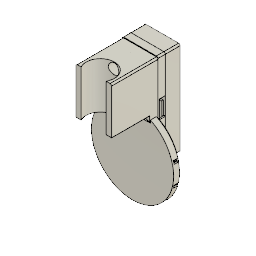
Wall Case v1 (Autodesk Fusion 360 design; units mm, degrees)
Autodesk Fusion 360 part; units mm, degrees
note: some values were not read from the file. Chosen so that the rebuilt part matches the saved one: which face or edge a step refers to. Set by a fixed rule: which sketch regions a step uses.
sketch "Bottom" plane through (0, 0, 0) normal (0, 0, 1) x (1, 0, 0) in component "Coil Case"
  arc A0 (33.9349, 0) -> (34.9349, 1) centre (33.9349, 1) ccw
  arc A1 (34.9349, 23) -> (33.9349, 24) centre (33.9349, 23) ccw
  line L0 (3.9349, 24) -> (3.9349, 0)
  circle A2 centre (30.9349, 12) radius 3.5
  circle A3 centre (30.9349, 12) radius 2.5
  line L1 (0, 0) -> (33.9349, 0)
  line L2 (34.9349, 1) -> (34.9349, 23)
  line L3 (33.9349, 24) -> (0, 24)
  line L4 (30.9349, 12) -> (34.9349, 12) construction
  line L5 (0, 0) -> (0, 24) construction
  circle A4 centre (-23.5651, 12) radius 26.5
  line L6 (0, 12) -> (-23.5651, 12) construction
  circle A5 centre (-23.5651, 12) radius 25.5
  circle A6 centre (-23.5651, 12) radius 2.5
  line L7 (-23.5651, 12) -> (-23.5651, -14.5) construction
  line L8 (-17.5651, -13.8118) -> (-17.5651, -12.7841)
  line L9 (-15.5651, -13.2636) -> (-15.5651, -12.2126)
  line L10 (-29.5651, -13.8118) -> (-29.5651, -12.7841)
  line L11 (-31.5651, -13.2636) -> (-31.5651, -12.2126)
  dimension "d2" = 7
  dimension "d4" = 33.9349
  dimension "d6" = 5
  dimension "d8" = 4
  dimension "d9" = 22
  dimension "d10" = 1
  dimension "d11" = 1
  dimension "d21" = 12
  dimension "d22" = 33.9349
  dimension "d23" = 3.9349
  dimension "d27" = 53
  dimension "d28" = 23.5651
  dimension "d29" = 51
  dimension "d30" = 5
  dimension "d37" = 2
  dimension "d38" = 6
  dimension "d24" = 0
  dimension "d25" = 0
  dimension "d26" = 0
  dimension "d35" = 0
  measures "d2" diameter of A2
  measures "d4" distance of A1.end L3.end
  measures "d6" diameter of A3
  measures "d8" distance of A2.centre L4.end
  measures "d9" distance of A0.end A1.start
  measures "d10" radius of A0
  measures "d11" radius of A1
  measures "d21" distance of A2.centre L1
  measures "d22" distance of A0.start L1.start
  measures "d23" distance of L0 L5
  measures "d27" diameter of A4
  measures "d28" distance of L6.start A4.centre
  measures "d29" diameter of A5
  measures "d30" diameter of A6
  measures "d37" distance of L8 L9
  measures "d38" distance of L7 L8
extrude "Extrude1" add sketch "Bottom" along normal blind 5.5 contours A0 A1 L0 L1 L2 L3 | L0 L1 L3 A4 | A2 makes body 1 in component "Coil Case"
extrude "Extrude2" add sketch "Bottom" along normal blind 25.5 from surface at 5.5 contours A0 A1 L0 L1 L2 L3 bodies 1 in component "Coil Case"
sketch "Side" plane through (34.9349, 0, 0) normal (1, 0, 0) x (0, 1, 0) in component "Coil Case"
  line L0 (1, 0) -> (23, 0)
  line L1 (23, 0) -> (23, 31)
  line L2 (23, 31) -> (1, 31)
  line L3 (1, 31) -> (1, 0)
  line L4 (12, 0) -> (12, 17) construction
  line L5 (12, 17) -> (12, 26.5) construction
  circle A0 centre (12, 26.5) radius 9.5
  dimension "d17" = 17
  dimension "d18" = 9.5
  measures "d17" distance of L4.start L4.end
  measures "d18" distance of L4.end L5.end
extrude "Extrude3" cut sketch "Side" against normal blind 31 contours L2 A0 | L2 A0 bodies 1 in component "Coil Case"
extrude "Extrude4" add sketch "Bottom" along normal blind 1 contours A4 A5 L9 L11 | A4 A5 L8 L9 | A4 A5 L10 L11 | A4 A5 L8 L10 | A5 bodies 1 in component "Coil Case"
extrude "Extrude5" add sketch "Bottom" along normal blind 2 contours A4 A5 L9 L11 | A4 A5 L8 L9 | A4 A5 L10 L11 | A4 A5 L8 L10 bodies 1 in component "Coil Case"
extrude "Extrude6" cut sketch "Bottom" against normal up to surface (1 mm away) from surface at 2 contours A4 A5 L8 L9 | A4 A5 L10 L11 bodies 1 in component "Coil Case"
sketch "Bottom (2)" plane through (0, 0, 0) normal (0, 1, 0) x (-1, 0, 0) in component "Coil Top"
  circle A0 centre (0, 0) radius 26.575
  circle A1 centre (0, 0) radius 27.575
  line L0 (6, -25.8888) -> (6, -26.9143)
  line L1 (8, -26.389) -> (8, -25.3423)
  line L2 (0, 0) -> (0, -27.575) construction
  line L3 (-6, -25.8888) -> (-6, -26.9143)
  line L4 (-8, -26.389) -> (-8, -25.3423)
  line L5 (0, 0) -> (0, 27.575) construction
  line L6 (0, 0) -> (-27.575, 0) construction
  line L7 (-23, 0) -> (-23, 12)
  line L8 (-23, 12) -> (-24.827, 12)
  line L9 (-23, 0) -> (-23, -12)
  line L10 (-23, -12) -> (-24.827, -12)
  dimension "d17_1" = 53.15
  dimension "d18_1" = 55.15
  dimension "d29_1" = 6
  dimension "d30_1" = 2
  dimension "d1" = 0
  dimension "d3" = 0
  dimension "d5" = 0
  dimension "d7" = 0
  dimension "d47" = 12
  dimension "d48" = 12
  measures "d17_1" diameter of A0
  measures "d18_1" diameter of A1
  measures "d29_1" distance of L0 L2
  measures "d30_1" distance of L0 L1
  measures "d47" distance of L7.start L7.end
  measures "d48" distance of L7.start L9.end
extrude "Extrude4'" add sketch "Bottom (2)" along normal blind 1 separate body contours A0 L7 L8 L9 L10 | A0 A1 L4 L10 | A0 A1 L3 L4 | A0 A1 L0 L3 | A0 A1 L0 L1 | A0 A1 L1 L8 picked at (9.9525, 1.3107) makes body 2 in component "Coil Top"
extrude "Extrude5'" add sketch "Bottom (2)" along normal blind 4 contours A0 A1 L4 L10 | A0 A1 L0 L3 | A0 A1 L1 L8 bodies 2 in component "Coil Top"
sketch "Bottom (3)" plane through (0, 0, 0) normal (0, 1, 0) x (-1, 0, 0) in component "PCB Top"
  arc A0 (-1, -24) -> (0, -23) centre (-1, -23) ccw
  line L0 (0, -23) -> (0, -1)
  arc A1 (0, -1) -> (-1, 0) centre (-1, -1) ccw
  line L1 (-63, -23) -> (-63, -1)
  line L2 (0, -1) -> (0, -23)
  arc A2 (-1, -24) -> (0, -23) centre (-1, -23) ccw
  arc A3 (-63, -23) -> (-62, -24) centre (-62, -23) ccw
  arc A4 (-62, 0) -> (-63, -1) centre (-62, -1) ccw
  arc A5 (0, -1) -> (-1, 0) centre (-1, -1) ccw
  circle A6 centre (-59, -12) radius 2.35
  circle A7 centre (-59, -12) radius 1.75
  circle A8 centre (-4, -12) radius 2.35
  circle A9 centre (-4, -12) radius 1.75
  line L3 (-1, -24) -> (-62, -24)
  line L4 (-9.2, -22.7) -> (-9.2, -18.7)
  line L5 (-9.2, -18.7) -> (-11.8, -18.7)
  line L6 (-11.8, -18.7) -> (-11.8, -22.7)
  line L7 (-11.8, -22.7) -> (-25.7, -22.7)
  line L8 (-25.7, -22.7) -> (-25.7, -22.5907)
  line L9 (-25.7, -22.5907) -> (-25.7, -18.7)
  line L10 (-25.7, -18.7) -> (-28.3, -18.7)
  line L11 (-28.3, -18.7) -> (-28.3, -22.7)
  line L12 (-28.3, -22.7) -> (-54.7, -22.7)
  line L13 (-54.7, -22.7) -> (-54.7, -3)
  arc A10 (-54, -2.3) -> (-54.7, -3) centre (-54, -3) ccw
  line L14 (-54, -2.3) -> (-37.3, -2.3)
  line L15 (-37.3, -4.8) -> (-37.3, -2.3)
  line L16 (-24.7, -4.8) -> (-37.3, -4.8)
  line L17 (-24.7, -2.3) -> (-24.7, -4.8)
  line L18 (-24.7, -2.3) -> (-9, -2.3)
  arc A11 (-8.3, -3) -> (-9, -2.3) centre (-9, -3) ccw
  line L19 (-8.3, -3) -> (-8.3, -22.7)
  line L20 (-8.3, -22.7) -> (-9.2, -22.7)
  line L21 (-4, -12) -> (0, -12) construction
  line L22 (-4, -12) -> (-4, 0) construction
  line L23 (-59, -12) -> (-59, 0) construction
  line L24 (-59, -12) -> (-63, -12) construction
  line L25 (-1, 0) -> (-62, 0)
  line L26 (0, 0) -> (-1, 0) construction
  line L27 (0, 0) -> (0, -1) construction
  dimension "d55_1" = 1
  dimension "d61" = 4.7
  dimension "d62" = 3.5
  dimension "d64" = 4.7
  dimension "d65" = 3.5
  dimension "d80" = 12
  dimension "d81" = 4
  dimension "d82" = 61
  dimension "d84" = 22
  dimension "d85" = 12
  dimension "d86" = 4
  dimension "d87" = 61
  dimension "d88" = 1
  dimension "d89" = 2.3
  dimension "d90" = 2.5
  dimension "d91" = 12.6
  dimension "d92" = 2.5
  dimension "d93" = 16.7
  dimension "d94" = 19.7
  dimension "d95" = 0.9
  dimension "d96" = 2.6
  dimension "d97" = 4
  dimension "d98" = 4
  dimension "d99" = 13.9
  dimension "d100" = 3.8907
  dimension "d101" = 2.6
  dimension "d102" = 4
  dimension "d103" = 26.4
  dimension "d104" = 19.7
  dimension "d105" = 0.7
  dimension "d106" = 8.3
  measures "d55_1" radius of A2
  measures "d61" diameter of A6
  measures "d62" diameter of A7
  measures "d64" diameter of A8
  measures "d65" diameter of A9
  measures "d80" distance of A8.centre L22.end
  measures "d81" distance of A8.centre L21.end
  measures "d82" distance of A3.end A0.start
  measures "d84" distance of L1.start L1.end
  measures "d85" distance of A6.centre L23.end
  measures "d86" distance of A6.centre L24.end
  measures "d87" distance of A4.start A1.end
  measures "d88" distance of A1.end L26.start
  measures "d89" distance of L18 L25
  measures "d90" distance of L16.start L17.start
  measures "d91" distance of L15.start L16.start
  measures "d92" distance of L14.end L15.start
  measures "d93" distance of A10.start L14.end
  measures "d94" distance of A11.start L19.end
  measures "d95" distance of L4.start L19.end
  measures "d96" distance of L4.end L5.end
  measures "d97" distance of L4.start L4.end
  measures "d98" distance of L5.end L6.end
  measures "d99" distance of L6.end L7.end
  measures "d100" distance of L8.end L9.end
  measures "d101" distance of L9.end L10.end
  measures "d102" distance of L10.end L11.end
  measures "d103" distance of L11.end L12.end
  measures "d104" distance of L12.end L13.end
  measures "d105" radius of A10
  measures "d106" distance of L2 L19
extrude "Extrude15" add sketch "Bottom (3)" along normal blind 10 separate body contours A0 L0 A1 L1 L2 A2 A3 A4 A5 L3 L25 | A6 | A8 | L4 L5 L6 L7 L8 L9 L10 L11 L12 L13 A10 L14 L15 L16 L17 L18 A11 L19 L20 makes body 3 in component "PCB Top"
extrude "Extrude16" add sketch "Bottom (3)" along normal blind 1 from surface at 10 contours L4 L5 L6 L7 L8 L9 L10 L11 L12 L13 A10 L14 L15 L16 L17 L18 A11 L19 L20 bodies 3 in component "PCB Top"
extrude "Extrude17" add sketch "Bottom (3)" along normal blind 2.5 from surface at 10 contours A6 | A8 bodies 3 in component "PCB Top"
sketch "Bottom (4)" plane through (0, 0, 0) normal (0, 1, 0) x (1, 0, 0) in component "PCB Bottom"
  line L0 (63, 1) -> (63, 23)
  arc A0 (63, 23) -> (62, 24) centre (62, 23) ccw
  arc A1 (62, 0) -> (63, 1) centre (62, 1) ccw
  line L1 (1, 0) -> (62, 0)
  line L2 (8, 23) -> (55, 23)
  circle A2 centre (59, 12) radius 2.5
  line L3 (62, 24) -> (1, 24)
  line L4 (0, 23) -> (0, 1)
  arc A3 (1, 24) -> (0, 23) centre (1, 23) ccw
  arc A4 (0, 1) -> (1, 0) centre (1, 1) ccw
  circle A5 centre (4, 12) radius 2.5
  line L5 (8, 23) -> (8, 3)
  line L6 (55, 23) -> (55, 3)
  line L7 (9, 2) -> (24, 2)
  line L8 (54, 2) -> (54, 2)
  line L9 (54, 2) -> (38, 2)
  line L10 (25, 1) -> (25, 0)
  line L11 (37, 1) -> (37, 0)
  arc A6 (8, 3) -> (9, 2) centre (9, 3) ccw
  arc A7 (25, 1) -> (24, 2) centre (24, 1) ccw
  arc A8 (38, 2) -> (37, 1) centre (38, 1) ccw
  arc A9 (54, 2) -> (55, 3) centre (54, 3) ccw
  line L12 (4, 12) -> (4, 0) construction
  line L13 (4, 12) -> (0, 12) construction
  line L14 (59, 12) -> (59, 0) construction
  line L15 (59, 12) -> (63, 12) construction
  line L16 (9.5, 23) -> (9.5, 24)
  line L17 (11.5, 23) -> (11.5, 24)
  line L18 (26, 23) -> (26, 24)
  line L19 (28, 23) -> (28, 24)
  point P0 (63, 0)
  point P1 (0, 24)
  point P2 (8, 2)
  point P3 (55, 2)
  point P4 (25, 2)
  point P5 (37, 2)
  dimension "d1_1" = 24
  dimension "d2_1" = 63
  dimension "d4_1" = 1
  dimension "d5_1" = 1
  dimension "d22_2" = 5
  dimension "d36_1" = 1
  dimension "d37_1" = 5
  dimension "d44_1" = 21
  dimension "d45" = 21
  dimension "d46" = 17
  dimension "d47_1" = 17
  dimension "d48_1" = 1
  dimension "d55_2" = 12
  dimension "d56_1" = 4
  dimension "d57" = 22
  dimension "d58" = 4
  dimension "d59" = 12
  dimension "d60" = 1
  dimension "d67" = 9.5
  dimension "d71" = 2
  dimension "d72" = 14.5
  dimension "d73" = 2
  measures "d1_1" distance of origin P1
  measures "d2_1" distance of origin P0
  measures "d4_1" radius of A0
  measures "d5_1" radius of A1
  measures "d22_2" diameter of A2
  measures "d36_1" radius of A3
  measures "d37_1" diameter of A5
  measures "d44_1" distance of L2.start P2
  measures "d45" distance of L2.end P3
  measures "d46" distance of P2 P4
  measures "d47_1" distance of L8.start P5
  measures "d48_1" radius of A6
  measures "d55_2" distance of A5.centre L12.end
  measures "d56_1" distance of A5.centre L13.end
  measures "d57" distance of L0.end L0.start
  measures "d58" distance of A2.centre L15.end
  measures "d59" distance of A2.centre L14.end
  measures "d60" distance of L2 L3
  measures "d67" distance of L4 L16
  measures "d71" distance of L16 L17
  measures "d72" distance of L17 L18
  measures "d73" distance of L18 L19
extrude "Extrude11" add sketch "Bottom (4)" along normal blind 1 separate body makes body 4 in component "PCB Bottom"
extrude "Extrude12" add sketch "Bottom (4)" along normal blind 5 contours L0 A0 A1 L1 L2 L3 L6 L9 L11 A8 A9 L19 | L2 L3 L18 L19 | L1 L2 L3 L4 A3 A4 L5 L7 L10 A6 A7 L16 | L2 L3 L17 L18 | L2 L3 L16 L17 bodies 4 in component "PCB Bottom"
extrude "Extrude13" cut sketch "Bottom (4)" against normal blind 3 from surface at 5 contours L2 L3 L18 L19 | L2 L3 L16 L17 bodies 4 in component "PCB Bottom"
component "Coil Case" placed x (0, 0, 1) y (-1, 0, 0) z (0, -1, 0) at (11.3814, 19.8844, 8.503)
component "Coil Top" placed x (0, 0, 1) y (0, 1, 0) z (-1, 0, 0) at (-0.6186, 14.8844, -15.0621)
component "PCB Top" placed x (0, 0, -1) y (0, -1, 0) z (-1, 0, 0) at (-12.6186, 34.8844, 43.9379)
component "PCB Bottom" placed x (0, 0, -1) y (0, 1, 0) z (1, 0, 0) at (11.3814, 19.8844, 43.9379)
equation "d22 = d4"
named bodies: "Wall", "Top", "PCB"
